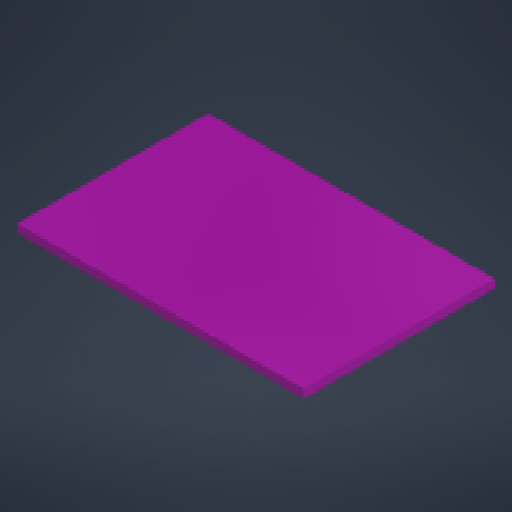
# Autodesk Inventor part: Chassi_inf
Saved by Autodesk Inventor 2026 (Build 300175000, 175)
## iProperties
Created: 2025-11-06
Part Number: Chassi_inf
Material: Genérico
Document SubType Name: Modeling
Designer: pregu
Density: 1 g/cm^3
Appearance: Suave - Púrpura
Author: pregu
Autodesk Inventor part; units mm, degrees
ref_plane "YZ Plane" through (0, 0, 0) normal (1, 0, 0) x (0, 1, 0)
ref_plane "XZ Plane" through (0, 0, 0) normal (0, 1, 0) x (-1, 0, 0)
ref_plane "XY Plane" through (0, 0, 0) normal (0, 0, 1) x (1, 0, 0)
sketch "Esboço1" plane through (0, 0, 0) normal (0, 1, 0) x (-1, 0, 0)
  line L0 (51.75, 50.222) -> (-51.75, 50.222)
  line L1 (51.75, 50.222) -> (-51.75, -50.222) construction
  line L2 (-51.75, 50.222) -> (51.75, -50.222) construction
  line L3 (-51.75, 50.222) -> (-51.75, -23.9989)
  line L4 (-38.75, -23.9989) -> (38.75, -23.9989)
  line L5 (51.75, -23.9989) -> (51.75, 50.222)
  line L6 (-46, 44.4719) -> (46, 44.4719) projected
  line L7 (-38.75, -23.9989) -> (-38.75, -48.7781)
  line L8 (-38.75, -56.7781) -> (-51.75, -56.7781)
  line L9 (-51.75, -56.7781) -> (-51.75, -23.9989)
  line L10 (46, -51.5281) -> (-46, -51.5281) projected
  line L11 (-38.75, -56.7781) -> (51.75, -56.7781)
  line L12 (51.75, -56.7781) -> (51.75, -48.7781)
  line L13 (38.75, -23.9989) -> (38.75, -48.7781)
  line L14 (51.75, -56.7781) -> (51.75, -23.9989)
  line L15 (51.75, -48.7781) -> (50.2621, -48.7781)
  line L16 (38.75, -48.7781) -> (-38.75, -48.7781)
  point P0 (0, 0)
  point P1 (0, 50.222)
  dimension "d3" = 103.5
  dimension "d7" = 51.75
  dimension "d13" = 50.222
  dimension "d16" = 13
  dimension "d17" = 5.25
  dimension "d18" = 8
  constraints: 30 end point, 4 parallel, 3 midpoint, 2 horizontal, 2 perpendicular, 2 vertical, 1 point on line
  measures "d3" distance of L0.start L0.end
  measures "d7" distance from line of L3 point (0, 0)
  measures "d13" distance from line of point (0, 0) L0
  measures "d16" distance of L8.start L8.end
  measures "d17" distance between parallel lines of L8 L10
  measures "d18" distance of L11.end L12.end
extrude "Extrusão1" add sketch "Esboço1" along normal blind 3
sketch "Esboço3" plane through (0, 0, 0) normal (0, -1, 0) x (1, 0, 0)
  line L0 (47.25, 28.672) -> (50.25, 28.672) projected
  line L1 (50.25, 28.672) -> (50.25, 40.672) projected
  line L2 (50.25, 40.672) -> (47.25, 40.672) projected
  line L3 (47.25, 28.672) -> (47.25, 40.672) projected
  line L4 (47.25, 7.122) -> (50.25, 7.122) projected
  line L5 (50.25, 7.122) -> (50.25, 19.122) projected
  line L6 (50.25, 19.122) -> (47.25, 19.122) projected
  line L7 (47.25, 7.122) -> (47.25, 19.122) projected
  line L8 (34.625, 45.7219) -> (34.625, 48.7219) projected
  line L9 (22.625, 48.7219) -> (34.625, 48.7219) projected
  line L10 (22.625, 48.7219) -> (22.625, 45.7219) projected
  line L11 (22.625, 45.7219) -> (34.625, 45.7219) projected
  line L12 (-6, 48.7219) -> (-6, 45.7219) projected
  line L13 (-6, 45.7219) -> (6, 45.7219) projected
  line L14 (6, 45.7219) -> (6, 48.7219) projected
  line L15 (-6, 48.7219) -> (6, 48.7219) projected
  line L16 (50.25, -2.428) -> (47.25, -2.428) projected
  line L17 (47.25, -14.428) -> (47.25, -2.428) projected
  line L18 (47.25, -14.428) -> (50.25, -14.428) projected
  line L19 (50.25, -14.428) -> (50.25, -2.428) projected
  line L20 (-22.625, 45.7219) -> (-22.625, 48.7219) projected
  line L21 (-34.625, 48.7219) -> (-22.625, 48.7219) projected
  line L22 (-34.625, 48.7219) -> (-34.625, 45.7219) projected
  line L23 (-34.625, 45.7219) -> (-22.625, 45.7219) projected
  line L24 (-34.625, 48.7219) -> (-22.625, 48.7219)
  line L25 (-22.625, 48.7219) -> (-22.625, 45.7219)
  line L26 (-22.625, 45.7219) -> (-34.625, 45.7219)
  line L27 (-34.625, 45.7219) -> (-34.625, 48.7219)
  line L28 (-6, 48.7219) -> (6, 48.7219)
  line L29 (6, 48.7219) -> (6, 45.7219)
  line L30 (6, 45.7219) -> (-6, 45.7219)
  line L31 (-6, 45.7219) -> (-6, 48.7219)
  line L32 (22.625, 48.7219) -> (34.625, 48.7219)
  line L33 (34.625, 48.7219) -> (34.625, 45.7219)
  line L34 (34.625, 45.7219) -> (22.625, 45.7219)
  line L35 (22.625, 45.7219) -> (22.625, 48.7219)
  line L36 (47.25, 40.672) -> (50.25, 40.672)
  line L37 (50.25, 40.672) -> (50.25, 28.672)
  line L38 (50.25, 28.672) -> (47.25, 28.672)
  line L39 (47.25, 28.672) -> (47.25, 40.672)
  line L40 (47.25, 19.122) -> (50.25, 19.122)
  line L41 (50.25, 19.122) -> (50.25, 7.122)
  line L42 (50.25, 7.122) -> (47.25, 7.122)
  line L43 (47.25, 7.122) -> (47.25, 19.122)
  line L44 (47.25, -2.428) -> (50.25, -2.428)
  line L45 (50.25, -2.428) -> (50.25, -14.428)
  line L46 (50.25, -14.428) -> (47.25, -14.428)
  line L47 (47.25, -14.428) -> (47.25, -2.428)
  line L48 (0, 54.2652) -> (0, -54.2652) construction
  line L49 (-47.25, 28.672) -> (-50.25, 28.672)
  line L50 (-50.25, 28.672) -> (-50.25, 40.672)
  line L51 (-50.25, 40.672) -> (-47.25, 40.672)
  line L52 (-47.25, 28.672) -> (-47.25, 40.672)
  line L53 (-47.25, 7.122) -> (-50.25, 7.122)
  line L54 (-50.25, 7.122) -> (-50.25, 19.122)
  line L55 (-50.25, 19.122) -> (-47.25, 19.122)
  line L56 (-47.25, 7.122) -> (-47.25, 19.122)
  line L57 (-50.25, -2.428) -> (-47.25, -2.428)
  line L58 (-47.25, -14.428) -> (-47.25, -2.428)
  line L59 (-47.25, -14.428) -> (-50.25, -14.428)
  line L60 (-50.25, -14.428) -> (-50.25, -2.428)
  line L61 (-47.25, 40.672) -> (-50.25, 40.672)
  line L62 (-50.25, 40.672) -> (-50.25, 28.672)
  line L63 (-50.25, 28.672) -> (-47.25, 28.672)
  line L64 (-47.25, 28.672) -> (-47.25, 40.672)
  line L65 (-47.25, 19.122) -> (-50.25, 19.122)
  line L66 (-50.25, 19.122) -> (-50.25, 7.122)
  line L67 (-50.25, 7.122) -> (-47.25, 7.122)
  line L68 (-47.25, 7.122) -> (-47.25, 19.122)
  line L69 (-47.25, -2.428) -> (-50.25, -2.428)
  line L70 (-50.25, -2.428) -> (-50.25, -14.428)
  line L71 (-50.25, -14.428) -> (-47.25, -14.428)
  line L72 (-47.25, -14.428) -> (-47.25, -2.428)
  point P0 (50.25, 25.222)
  point P1 (47.25, 37.222)
  point P2 (0, 0)
  point P3 (-50.25, 25.222)
  point P4 (-47.25, 37.222)
  constraints: 98 end point, 20 symmetric about line, 12 parallel, 6 horizontal, 6 perpendicular, 1 midpoint, 1 vertical
extrude "Extrusão3" cut sketch "Esboço3" against normal blind 3
equation "\"d7\" = 0.5 * d3"
